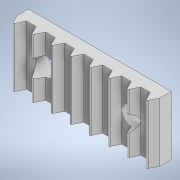
# Autodesk Inventor part: time belt coupling
Saved by Autodesk Inventor 2021 (Build 250183000, 183)
## iProperties
Created: 2021-04-19
Part Number: time belt coupling
Material: Generic
Document SubType Name: Modeling
Designer: Olivi
Density: 1 g/cm^3
Appearance: Default
Author: Olivi
Autodesk Inventor part; units mm, degrees
ref_plane "YZ Plane" through (0, 0, 0) normal (1, 0, 0) x (0, 1, 0)
ref_plane "XZ Plane" through (0, 0, 0) normal (0, 1, 0) x (-1, 0, 0)
ref_plane "XY Plane" through (0, 0, 0) normal (0, 0, 1) x (1, 0, 0)
sketch "Sketch1" plane through (0, 0, 0) normal (0, 0, 1) x (1, 0, 0)
  line L0 (0, 0) -> (0, 6.2)
  line L1 (0, 6.2) -> (15, 6.2)
  line L2 (15, 6.2) -> (15, 0)
  line L3 (15, 0) -> (0, 0)
  dimension "d0" = 6.2
  dimension "d1" = 15
  constraints: 8 end point, 3 perpendicular, 1 vertical
  measures "d0" distance of L0.start L0.end
  measures "d1" distance of L0.end L1.end
extrude "Extrusion1" add sketch "Sketch1" along normal blind 1.2
sketch "Sketch2" plane through (0, 0, 0) normal (0, -1, 0) x (1, 0, 0)
  line L0 (0, 0) -> (0, 1.2) projected
  line L1 (0, 1.2) -> (0.5, 1.2)
  line L2 (15, 1.2) -> (0, 1.2) projected
  line L3 (0.5, 1.2) -> (0.5, 2.2)
  line L4 (0.5, 2.2) -> (0, 1.2)
  line L5 (0.5, 1.2) -> (1, 1.2)
  line L6 (1, 1.2) -> (0.5, 2.2)
  dimension "d4" = 0.5
  dimension "d5" = 1
  dimension "d6" = 0.5
  constraints: 10 end point, 2 point on line, 1 perpendicular
  measures "d4" distance of L0.end L1.end
  measures "d5" distance of L1.end L3.end
  measures "d6" distance of L1.end L5.end
extrude "Extrusion2" add sketch "Sketch2" against normal blind 6.2
fillet "Fillet1" radius 0.1 1 edges at (0.5, 3.1, 2.2)
pattern_linear "Rectangular Pattern1" count 8 spacing 2 along (1, 0, 0) of "Fillet1", "Extrusion2"
sketch "Sketch3" plane through (0, 0, 0) normal (0, 0, -1) x (-1, 0, 0)
  circle A0 centre (-3, 3.1) radius 1
  circle A1 centre (-12, 3.1) radius 1
  line L0 (0, 6.2) -> (0, 0) projected
  line L1 (-15, 0) -> (-15, 6.2) projected
  dimension "d13" = 2
  dimension "d14" = 2
  dimension "d15" = 3
  dimension "d16" = 3
  constraints: 2 centre point
  measures "d13" diameter of A0
  measures "d14" diameter of A1
  measures "d15" distance from line of L0 A0.centre
  measures "d16" distance from line of L1 A1.centre
extrude "Extrusion3" cut sketch "Sketch3" against normal blind 6.2
body "Solid1"
